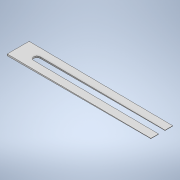
# Autodesk Inventor part: WinderSpoolRemovalAid
Saved by Autodesk Inventor 2022 (Build 260153070, 153G)
## iProperties
Created: 2021-05-24
Part Number: WinderSpoolRemovalAid
Material: Generic
Document SubType Name: Modeling
Designer: elmar
Density: 1 g/cm^3
Appearance: Default
Author: elmar
Autodesk Inventor part; units mm, degrees
ref_plane "YZ Plane" through (0, 0, 0) normal (1, 0, 0) x (0, 1, 0)
ref_plane "XZ Plane" through (0, 0, 0) normal (0, 1, 0) x (-1, 0, 0)
ref_plane "XY Plane" through (0, 0, 0) normal (0, 0, 1) x (1, 0, 0)
sketch "Sketch1" plane through (0, 0, 0) normal (0, 0, 1) x (1, 0, 0)
  line L0 (0, 0) -> (0, 0.5)
  line L1 (0, 0.5) -> (-230, 2.5909)
  line L2 (-230, 2.5909) -> (-230, 0)
  line L3 (-230, 0) -> (0, 0)
  line L4 (-55, 0) -> (-55, 1)
  dimension "d0" = 55
  dimension "d1" = 1
  dimension "d2" = 0.5
  dimension "d10" = 230
  constraints: 10 end point, 2 point on line, 2 vertical, 1 parallel, 1 perpendicular
  measures "d0" distance of L0.start L4.start
  measures "d1" distance of L4.start L4.end
  measures "d2" distance of L0.start L0.end
  measures "d10" distance between parallel lines of L0 L2
extrude "Extrusion1" add sketch "Sketch1" along normal blind 35
sketch "Sketch2" plane through (-230, 0, 0) normal (0, -1, 0) x (1, 0, 0)
  line L0 (230, 0) -> (230, 35) projected
  line L1 (230, 17.5) -> (30, 17.5) construction
  line L2 (230, 12.3) -> (30, 12.3)
  line L3 (30, 22.7) -> (230, 22.7)
  arc A0 (230, 12.3) -> (230, 22.7) centre (230, 17.5) ccw
  arc A1 (30, 22.7) -> (30, 12.3) centre (30, 17.5) ccw
  point P0 (130, 17.5)
  dimension "d6" = 200
  dimension "d7" = 5.2
  constraints: 8 end point, 4 point on circle, 4 tangent, 2 centre point, 2 midpoint, 1 parallel, 1 perpendicular
  measures "d6" distance of L1.start L1.end
  measures "d7" radius of A1
extrude "Extrusion2" cut sketch "Sketch2" against normal through all contours L2 A1 L3 L0
body "Solid1"
